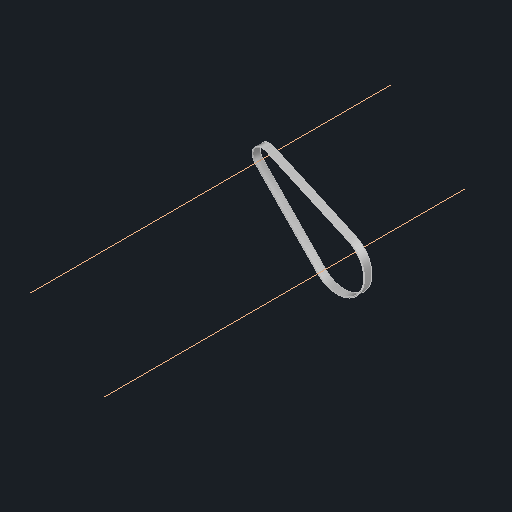
# Autodesk Inventor part: Synchronous Belt
Saved by Autodesk Inventor 2025.2 (Build 292293000, 293)
## iProperties
Created: 2025-05-28
Part Number: Synchronous Belt
Material: Rubber
Document SubType Name: Modeling
Designer: Tiago
Density: 1 g/cm^3
Appearance: Rubber - Black - Version 1.1
CustomPartVersion: 1
Author: Tiago
Autodesk Inventor part; units mm, degrees
sketch "Sketch Path" plane through (0, 0, 0) normal (0, 0, 1) x (1, 0, 0)
  arc A0 (10.7065, 10.1475) -> (1.7608, -2.6697) centre (7.4634, 2.8807) ccw
  arc A1 (52.3809, -54.6782) -> (76.9817, -19.4308) centre (68.063, -39.4147) ccw
  line L0 (52.3809, -54.6782) -> (1.7608, -2.6697)
  line L1 (10.7065, 10.1475) -> (76.9817, -19.4308)
  constraints: 4 end point, 4 point on circle, 2 centre point
ref_plane "Cross Section Plane" through (1.7608, -2.6697, 0) normal (0.6975, -0.7166, 0) x (0, 0, 1)
ref_plane "Work Plane2" through (7.4634, 2.8807, 0) normal (-1, 0, 0) x (0, 0, 1)
ref_plane "Work Plane3" through (68.063, -39.4147, 0) normal (-0.8813, 0.4725, 0) x (0, 0, 1)
sketch "Cross Section" plane through (1.7608, -2.6697, 0) normal (0.6975, -0.7166, 0) x (0, 0, 1)
  line L0 (-3, 0.3) -> (3, 0.3)
  line L1 (3, 0.3) -> (3, -0.3)
  line L2 (3, -0.3) -> (-3, -0.3)
  line L3 (-3, -0.3) -> (-3, 0.3)
  line L4 (-3, 0) -> (3, 0) construction
  point P0 (0, 0)
  point P1 (0, 0)
  dimension "d0" = 6
  dimension "d4" = 0.3
  dimension "d5" = 0.3
  constraints: 10 end point, 3 midpoint, 2 parallel, 1 coincident, 1 horizontal, 1 perpendicular, 1 other
  measures "d0" distance between parallel lines of L1 L3
  measures "d4" distance between parallel lines of L2 L4
  measures "d5" distance between parallel lines of L4 L0
sweep "Belt" add profiles "Cross Section" path "Sketch Path"
equation "\"d0\" = da_B"
equation "\"d4\" = da_a"
equation "\"d5\" = da_a2"
equation "\"da_B\" = 6"
equation "\"da_pb\" = 2.5"
equation "\"da_L\" = 244.18214"
equation "\"da_a\" = 0.3"
equation "\"da_S\" = 1.5"
equation "\"da_Beta\" = 20deg"
equation "\"da_Ht\" = 0.7"
equation "\"da_H\" = 1.3"
equation "\"da_a2\" = 0.3"
body "Solid1"
